Autodesk Fusion 360 part; units mm, degrees
(part 2 of 2)
  circle A962 centre (86.8214, 134.766) radius 1.25
  circle A963 centre (91.2857, 134.766) radius 1.25
  circle A964 centre (95.75, 134.766) radius 1.25
  circle A965 centre (100.2143, 134.766) radius 1.25
  circle A966 centre (104.6786, 134.766) radius 1.25
  circle A967 centre (109.1429, 134.766) radius 1.25
  circle A968 centre (113.6071, 134.766) radius 1.25
  circle A969 centre (118.0714, 134.766) radius 1.25
  circle A970 centre (122.5357, 134.766) radius 1.25
  circle A971 centre (127, 134.766) radius 1.25
  circle A972 centre (42.1786, 139.8723) radius 1.25
  circle A973 centre (46.6429, 139.8723) radius 1.25
  circle A974 centre (51.1071, 139.8723) radius 1.25
  circle A975 centre (55.5714, 139.8723) radius 1.25
  circle A976 centre (60.0357, 139.8723) radius 1.25
  circle A977 centre (64.5, 139.8723) radius 1.25
  circle A978 centre (68.9643, 139.8723) radius 1.25
  circle A979 centre (73.4286, 139.8723) radius 1.25
  circle A980 centre (77.8929, 139.8723) radius 1.25
  circle A981 centre (82.3571, 139.8723) radius 1.25
  circle A982 centre (86.8214, 139.8723) radius 1.25
  circle A983 centre (91.2857, 139.8723) radius 1.25
  circle A984 centre (95.75, 139.8723) radius 1.25
  circle A985 centre (100.2143, 139.8723) radius 1.25
  circle A986 centre (104.6786, 139.8723) radius 1.25
  circle A987 centre (109.1429, 139.8723) radius 1.25
  circle A988 centre (113.6071, 139.8723) radius 1.25
  circle A989 centre (118.0714, 139.8723) radius 1.25
  circle A990 centre (122.5357, 139.8723) radius 1.25
  circle A991 centre (127, 139.8723) radius 1.25
  circle A992 centre (42.1786, 144.9787) radius 1.25
  circle A993 centre (46.6429, 144.9787) radius 1.25
  circle A994 centre (51.1071, 144.9787) radius 1.25
  circle A995 centre (55.5714, 144.9787) radius 1.25
  circle A996 centre (60.0357, 144.9787) radius 1.25
  circle A997 centre (64.5, 144.9787) radius 1.25
  circle A998 centre (68.9643, 144.9787) radius 1.25
  circle A999 centre (73.4286, 144.9787) radius 1.25
  circle A1000 centre (77.8929, 144.9787) radius 1.25
  circle A1001 centre (82.3571, 144.9787) radius 1.25
  circle A1002 centre (86.8214, 144.9787) radius 1.25
  circle A1003 centre (91.2857, 144.9787) radius 1.25
  circle A1004 centre (95.75, 144.9787) radius 1.25
  circle A1005 centre (100.2143, 144.9787) radius 1.25
  circle A1006 centre (104.6786, 144.9787) radius 1.25
  circle A1007 centre (109.1429, 144.9787) radius 1.25
  circle A1008 centre (113.6071, 144.9787) radius 1.25
  circle A1009 centre (118.0714, 144.9787) radius 1.25
  circle A1010 centre (122.5357, 144.9787) radius 1.25
  circle A1011 centre (127, 144.9787) radius 1.25
  circle A1012 centre (42.1786, 150.0851) radius 1.25
  circle A1013 centre (46.6429, 150.0851) radius 1.25
  circle A1014 centre (51.1071, 150.0851) radius 1.25
  circle A1015 centre (55.5714, 150.0851) radius 1.25
  circle A1016 centre (60.0357, 150.0851) radius 1.25
  circle A1017 centre (64.5, 150.0851) radius 1.25
  circle A1018 centre (68.9643, 150.0851) radius 1.25
  circle A1019 centre (73.4286, 150.0851) radius 1.25
  circle A1020 centre (77.8929, 150.0851) radius 1.25
  circle A1021 centre (82.3571, 150.0851) radius 1.25
  circle A1022 centre (86.8214, 150.0851) radius 1.25
  circle A1023 centre (91.2857, 150.0851) radius 1.25
  circle A1024 centre (95.75, 150.0851) radius 1.25
  circle A1025 centre (100.2143, 150.0851) radius 1.25
  circle A1026 centre (104.6786, 150.0851) radius 1.25
  circle A1027 centre (109.1429, 150.0851) radius 1.25
  circle A1028 centre (113.6071, 150.0851) radius 1.25
  circle A1029 centre (118.0714, 150.0851) radius 1.25
  circle A1030 centre (122.5357, 150.0851) radius 1.25
  circle A1031 centre (127, 150.0851) radius 1.25
  circle A1032 centre (42.1786, 155.1915) radius 1.25
  circle A1033 centre (46.6429, 155.1915) radius 1.25
  circle A1034 centre (51.1071, 155.1915) radius 1.25
  circle A1035 centre (55.5714, 155.1915) radius 1.25
  circle A1036 centre (60.0357, 155.1915) radius 1.25
  circle A1037 centre (64.5, 155.1915) radius 1.25
  circle A1038 centre (68.9643, 155.1915) radius 1.25
  circle A1039 centre (73.4286, 155.1915) radius 1.25
  circle A1040 centre (77.8929, 155.1915) radius 1.25
  circle A1041 centre (82.3571, 155.1915) radius 1.25
  circle A1042 centre (86.8214, 155.1915) radius 1.25
  circle A1043 centre (91.2857, 155.1915) radius 1.25
  circle A1044 centre (95.75, 155.1915) radius 1.25
  circle A1045 centre (100.2143, 155.1915) radius 1.25
  circle A1046 centre (104.6786, 155.1915) radius 1.25
  circle A1047 centre (109.1429, 155.1915) radius 1.25
  circle A1048 centre (113.6071, 155.1915) radius 1.25
  circle A1049 centre (118.0714, 155.1915) radius 1.25
  circle A1050 centre (122.5357, 155.1915) radius 1.25
  circle A1051 centre (127, 155.1915) radius 1.25
  circle A1052 centre (42.1786, 160.2979) radius 1.25
  circle A1053 centre (46.6429, 160.2979) radius 1.25
  circle A1054 centre (51.1071, 160.2979) radius 1.25
  circle A1055 centre (55.5714, 160.2979) radius 1.25
  circle A1056 centre (60.0357, 160.2979) radius 1.25
  circle A1057 centre (64.5, 160.2979) radius 1.25
  circle A1058 centre (68.9643, 160.2979) radius 1.25
  circle A1059 centre (73.4286, 160.2979) radius 1.25
  circle A1060 centre (77.8929, 160.2979) radius 1.25
  circle A1061 centre (82.3571, 160.2979) radius 1.25
  circle A1062 centre (86.8214, 160.2979) radius 1.25
  circle A1063 centre (91.2857, 160.2979) radius 1.25
  circle A1064 centre (95.75, 160.2979) radius 1.25
  circle A1065 centre (100.2143, 160.2979) radius 1.25
  circle A1066 centre (104.6786, 160.2979) radius 1.25
  circle A1067 centre (109.1429, 160.2979) radius 1.25
  circle A1068 centre (113.6071, 160.2979) radius 1.25
  circle A1069 centre (118.0714, 160.2979) radius 1.25
  circle A1070 centre (122.5357, 160.2979) radius 1.25
  circle A1071 centre (127, 160.2979) radius 1.25
  circle A1072 centre (42.1786, 165.4043) radius 1.25
  circle A1073 centre (46.6429, 165.4043) radius 1.25
  circle A1074 centre (51.1071, 165.4043) radius 1.25
  circle A1075 centre (55.5714, 165.4043) radius 1.25
  circle A1076 centre (60.0357, 165.4043) radius 1.25
  circle A1077 centre (64.5, 165.4043) radius 1.25
  circle A1078 centre (68.9643, 165.4043) radius 1.25
  circle A1079 centre (73.4286, 165.4043) radius 1.25
  circle A1080 centre (77.8929, 165.4043) radius 1.25
  circle A1081 centre (82.3571, 165.4043) radius 1.25
  circle A1082 centre (86.8214, 165.4043) radius 1.25
  circle A1083 centre (91.2857, 165.4043) radius 1.25
  circle A1084 centre (95.75, 165.4043) radius 1.25
  circle A1085 centre (100.2143, 165.4043) radius 1.25
  circle A1086 centre (104.6786, 165.4043) radius 1.25
  circle A1087 centre (109.1429, 165.4043) radius 1.25
  circle A1088 centre (113.6071, 165.4043) radius 1.25
  circle A1089 centre (118.0714, 165.4043) radius 1.25
  circle A1090 centre (122.5357, 165.4043) radius 1.25
  circle A1091 centre (127, 165.4043) radius 1.25
  circle A1092 centre (42.1786, 170.5106) radius 1.25
  circle A1093 centre (46.6429, 170.5106) radius 1.25
  circle A1094 centre (51.1071, 170.5106) radius 1.25
  circle A1095 centre (55.5714, 170.5106) radius 1.25
  circle A1096 centre (60.0357, 170.5106) radius 1.25
  circle A1097 centre (64.5, 170.5106) radius 1.25
  circle A1098 centre (68.9643, 170.5106) radius 1.25
  circle A1099 centre (73.4286, 170.5106) radius 1.25
  circle A1100 centre (77.8929, 170.5106) radius 1.25
  circle A1101 centre (82.3571, 170.5106) radius 1.25
  circle A1102 centre (86.8214, 170.5106) radius 1.25
  circle A1103 centre (91.2857, 170.5106) radius 1.25
  circle A1104 centre (95.75, 170.5106) radius 1.25
  circle A1105 centre (100.2143, 170.5106) radius 1.25
  circle A1106 centre (104.6786, 170.5106) radius 1.25
  circle A1107 centre (109.1429, 170.5106) radius 1.25
  circle A1108 centre (113.6071, 170.5106) radius 1.25
  circle A1109 centre (118.0714, 170.5106) radius 1.25
  circle A1110 centre (122.5357, 170.5106) radius 1.25
  circle A1111 centre (127, 170.5106) radius 1.25
  circle A1112 centre (42.1786, 175.617) radius 1.25
  circle A1113 centre (46.6429, 175.617) radius 1.25
  circle A1114 centre (51.1071, 175.617) radius 1.25
  circle A1115 centre (55.5714, 175.617) radius 1.25
  circle A1116 centre (60.0357, 175.617) radius 1.25
  circle A1117 centre (64.5, 175.617) radius 1.25
  circle A1118 centre (68.9643, 175.617) radius 1.25
  circle A1119 centre (73.4286, 175.617) radius 1.25
  circle A1120 centre (77.8929, 175.617) radius 1.25
  circle A1121 centre (82.3571, 175.617) radius 1.25
  circle A1122 centre (86.8214, 175.617) radius 1.25
  circle A1123 centre (91.2857, 175.617) radius 1.25
  circle A1124 centre (95.75, 175.617) radius 1.25
  circle A1125 centre (100.2143, 175.617) radius 1.25
  circle A1126 centre (104.6786, 175.617) radius 1.25
  circle A1127 centre (109.1429, 175.617) radius 1.25
  circle A1128 centre (113.6071, 175.617) radius 1.25
  circle A1129 centre (118.0714, 175.617) radius 1.25
  circle A1130 centre (122.5357, 175.617) radius 1.25
  circle A1131 centre (127, 175.617) radius 1.25
  circle A1132 centre (42.1786, 180.7234) radius 1.25
  circle A1133 centre (46.6429, 180.7234) radius 1.25
  circle A1134 centre (51.1071, 180.7234) radius 1.25
  circle A1135 centre (55.5714, 180.7234) radius 1.25
  circle A1136 centre (60.0357, 180.7234) radius 1.25
  circle A1137 centre (64.5, 180.7234) radius 1.25
  circle A1138 centre (68.9643, 180.7234) radius 1.25
  circle A1139 centre (73.4286, 180.7234) radius 1.25
  circle A1140 centre (77.8929, 180.7234) radius 1.25
  circle A1141 centre (82.3571, 180.7234) radius 1.25
  circle A1142 centre (86.8214, 180.7234) radius 1.25
  circle A1143 centre (91.2857, 180.7234) radius 1.25
  circle A1144 centre (95.75, 180.7234) radius 1.25
  circle A1145 centre (100.2143, 180.7234) radius 1.25
  circle A1146 centre (104.6786, 180.7234) radius 1.25
  circle A1147 centre (109.1429, 180.7234) radius 1.25
  circle A1148 centre (113.6071, 180.7234) radius 1.25
  circle A1149 centre (118.0714, 180.7234) radius 1.25
  circle A1150 centre (122.5357, 180.7234) radius 1.25
  circle A1151 centre (127, 180.7234) radius 1.25
  circle A1152 centre (42.1786, 185.8298) radius 1.25
  circle A1153 centre (46.6429, 185.8298) radius 1.25
  circle A1154 centre (51.1071, 185.8298) radius 1.25
  circle A1155 centre (55.5714, 185.8298) radius 1.25
  circle A1156 centre (60.0357, 185.8298) radius 1.25
  circle A1157 centre (64.5, 185.8298) radius 1.25
  circle A1158 centre (68.9643, 185.8298) radius 1.25
  circle A1159 centre (73.4286, 185.8298) radius 1.25
  circle A1160 centre (77.8929, 185.8298) radius 1.25
  circle A1161 centre (82.3571, 185.8298) radius 1.25
  circle A1162 centre (86.8214, 185.8298) radius 1.25
  circle A1163 centre (91.2857, 185.8298) radius 1.25
  circle A1164 centre (95.75, 185.8298) radius 1.25
  circle A1165 centre (100.2143, 185.8298) radius 1.25
  circle A1166 centre (104.6786, 185.8298) radius 1.25
  circle A1167 centre (109.1429, 185.8298) radius 1.25
  circle A1168 centre (113.6071, 185.8298) radius 1.25
  circle A1169 centre (118.0714, 185.8298) radius 1.25
  circle A1170 centre (122.5357, 185.8298) radius 1.25
  circle A1171 centre (127, 185.8298) radius 1.25
  circle A1172 centre (42.1786, 190.9362) radius 1.25
  circle A1173 centre (46.6429, 190.9362) radius 1.25
  circle A1174 centre (51.1071, 190.9362) radius 1.25
  circle A1175 centre (55.5714, 190.9362) radius 1.25
  circle A1176 centre (60.0357, 190.9362) radius 1.25
  circle A1177 centre (64.5, 190.9362) radius 1.25
  circle A1178 centre (68.9643, 190.9362) radius 1.25
  circle A1179 centre (73.4286, 190.9362) radius 1.25
  circle A1180 centre (77.8929, 190.9362) radius 1.25
  circle A1181 centre (82.3571, 190.9362) radius 1.25
  circle A1182 centre (86.8214, 190.9362) radius 1.25
  circle A1183 centre (91.2857, 190.9362) radius 1.25
  circle A1184 centre (95.75, 190.9362) radius 1.25
  circle A1185 centre (100.2143, 190.9362) radius 1.25
  circle A1186 centre (104.6786, 190.9362) radius 1.25
  circle A1187 centre (109.1429, 190.9362) radius 1.25
  circle A1188 centre (113.6071, 190.9362) radius 1.25
  circle A1189 centre (118.0714, 190.9362) radius 1.25
  circle A1190 centre (122.5357, 190.9362) radius 1.25
  circle A1191 centre (127, 190.9362) radius 1.25
  circle A1192 centre (42.1786, 196.0426) radius 1.25
  circle A1193 centre (46.6429, 196.0426) radius 1.25
  circle A1194 centre (51.1071, 196.0426) radius 1.25
  circle A1195 centre (55.5714, 196.0426) radius 1.25
  circle A1196 centre (60.0357, 196.0426) radius 1.25
  circle A1197 centre (64.5, 196.0426) radius 1.25
  circle A1198 centre (68.9643, 196.0426) radius 1.25
  circle A1199 centre (73.4286, 196.0426) radius 1.25
  circle A1200 centre (77.8929, 196.0426) radius 1.25
  circle A1201 centre (82.3571, 196.0426) radius 1.25
  circle A1202 centre (86.8214, 196.0426) radius 1.25
  circle A1203 centre (91.2857, 196.0426) radius 1.25
  circle A1204 centre (95.75, 196.0426) radius 1.25
  circle A1205 centre (100.2143, 196.0426) radius 1.25
  circle A1206 centre (104.6786, 196.0426) radius 1.25
  circle A1207 centre (109.1429, 196.0426) radius 1.25
  circle A1208 centre (113.6071, 196.0426) radius 1.25
  circle A1209 centre (118.0714, 196.0426) radius 1.25
  circle A1210 centre (122.5357, 196.0426) radius 1.25
  circle A1211 centre (127, 196.0426) radius 1.25
  circle A1212 centre (42.1786, 201.1489) radius 1.25
  circle A1213 centre (46.6429, 201.1489) radius 1.25
  circle A1214 centre (51.1071, 201.1489) radius 1.25
  circle A1215 centre (55.5714, 201.1489) radius 1.25
  circle A1216 centre (60.0357, 201.1489) radius 1.25
  circle A1217 centre (64.5, 201.1489) radius 1.25
  circle A1218 centre (68.9643, 201.1489) radius 1.25
  circle A1219 centre (73.4286, 201.1489) radius 1.25
  circle A1220 centre (77.8929, 201.1489) radius 1.25
  circle A1221 centre (82.3571, 201.1489) radius 1.25
  circle A1222 centre (86.8214, 201.1489) radius 1.25
  circle A1223 centre (91.2857, 201.1489) radius 1.25
  circle A1224 centre (95.75, 201.1489) radius 1.25
  circle A1225 centre (100.2143, 201.1489) radius 1.25
  circle A1226 centre (104.6786, 201.1489) radius 1.25
  circle A1227 centre (109.1429, 201.1489) radius 1.25
  circle A1228 centre (113.6071, 201.1489) radius 1.25
  circle A1229 centre (118.0714, 201.1489) radius 1.25
  circle A1230 centre (122.5357, 201.1489) radius 1.25
  circle A1231 centre (127, 201.1489) radius 1.25
  circle A1232 centre (42.1786, 206.2553) radius 1.25
  circle A1233 centre (46.6429, 206.2553) radius 1.25
  circle A1234 centre (51.1071, 206.2553) radius 1.25
  circle A1235 centre (55.5714, 206.2553) radius 1.25
  circle A1236 centre (60.0357, 206.2553) radius 1.25
  circle A1237 centre (64.5, 206.2553) radius 1.25
  circle A1238 centre (68.9643, 206.2553) radius 1.25
  circle A1239 centre (73.4286, 206.2553) radius 1.25
  circle A1240 centre (77.8929, 206.2553) radius 1.25
  circle A1241 centre (82.3571, 206.2553) radius 1.25
  circle A1242 centre (86.8214, 206.2553) radius 1.25
  circle A1243 centre (91.2857, 206.2553) radius 1.25
  circle A1244 centre (95.75, 206.2553) radius 1.25
  circle A1245 centre (100.2143, 206.2553) radius 1.25
  circle A1246 centre (104.6786, 206.2553) radius 1.25
  circle A1247 centre (109.1429, 206.2553) radius 1.25
  circle A1248 centre (113.6071, 206.2553) radius 1.25
  circle A1249 centre (118.0714, 206.2553) radius 1.25
  circle A1250 centre (122.5357, 206.2553) radius 1.25
  circle A1251 centre (127, 206.2553) radius 1.25
  circle A1252 centre (42.1786, 211.3617) radius 1.25
  circle A1253 centre (46.6429, 211.3617) radius 1.25
  circle A1254 centre (51.1071, 211.3617) radius 1.25
  circle A1255 centre (55.5714, 211.3617) radius 1.25
  circle A1256 centre (60.0357, 211.3617) radius 1.25
  circle A1257 centre (64.5, 211.3617) radius 1.25
  circle A1258 centre (68.9643, 211.3617) radius 1.25
  circle A1259 centre (73.4286, 211.3617) radius 1.25
  circle A1260 centre (77.8929, 211.3617) radius 1.25
  circle A1261 centre (82.3571, 211.3617) radius 1.25
  circle A1262 centre (86.8214, 211.3617) radius 1.25
  circle A1263 centre (91.2857, 211.3617) radius 1.25
  circle A1264 centre (95.75, 211.3617) radius 1.25
  circle A1265 centre (100.2143, 211.3617) radius 1.25
  circle A1266 centre (104.6786, 211.3617) radius 1.25
  circle A1267 centre (109.1429, 211.3617) radius 1.25
  circle A1268 centre (113.6071, 211.3617) radius 1.25
  circle A1269 centre (118.0714, 211.3617) radius 1.25
  circle A1270 centre (122.5357, 211.3617) radius 1.25
  circle A1271 centre (127, 211.3617) radius 1.25
  circle A1272 centre (42.1786, 216.4681) radius 1.25
  circle A1273 centre (46.6429, 216.4681) radius 1.25
  circle A1274 centre (51.1071, 216.4681) radius 1.25
  circle A1275 centre (55.5714, 216.4681) radius 1.25
  circle A1276 centre (60.0357, 216.4681) radius 1.25
  circle A1277 centre (64.5, 216.4681) radius 1.25
  circle A1278 centre (68.9643, 216.4681) radius 1.25
  circle A1279 centre (73.4286, 216.4681) radius 1.25
  circle A1280 centre (77.8929, 216.4681) radius 1.25
  circle A1281 centre (82.3571, 216.4681) radius 1.25
  circle A1282 centre (86.8214, 216.4681) radius 1.25
  circle A1283 centre (91.2857, 216.4681) radius 1.25
  circle A1284 centre (95.75, 216.4681) radius 1.25
  circle A1285 centre (100.2143, 216.4681) radius 1.25
  circle A1286 centre (104.6786, 216.4681) radius 1.25
  circle A1287 centre (109.1429, 216.4681) radius 1.25
  circle A1288 centre (113.6071, 216.4681) radius 1.25
  circle A1289 centre (118.0714, 216.4681) radius 1.25
  circle A1290 centre (122.5357, 216.4681) radius 1.25
  circle A1291 centre (127, 216.4681) radius 1.25
  circle A1292 centre (42.1786, 221.5745) radius 1.25
  circle A1293 centre (46.6429, 221.5745) radius 1.25
  circle A1294 centre (51.1071, 221.5745) radius 1.25
  circle A1295 centre (55.5714, 221.5745) radius 1.25
  circle A1296 centre (60.0357, 221.5745) radius 1.25
  circle A1297 centre (64.5, 221.5745) radius 1.25
  circle A1298 centre (68.9643, 221.5745) radius 1.25
  circle A1299 centre (73.4286, 221.5745) radius 1.25
  circle A1300 centre (77.8929, 221.5745) radius 1.25
  circle A1301 centre (82.3571, 221.5745) radius 1.25
  circle A1302 centre (86.8214, 221.5745) radius 1.25
  circle A1303 centre (91.2857, 221.5745) radius 1.25
  circle A1304 centre (95.75, 221.5745) radius 1.25
  circle A1305 centre (100.2143, 221.5745) radius 1.25
  circle A1306 centre (104.6786, 221.5745) radius 1.25
  circle A1307 centre (109.1429, 221.5745) radius 1.25
  circle A1308 centre (113.6071, 221.5745) radius 1.25
  circle A1309 centre (118.0714, 221.5745) radius 1.25
  circle A1310 centre (122.5357, 221.5745) radius 1.25
  circle A1311 centre (127, 221.5745) radius 1.25
  circle A1312 centre (42.1786, 226.6809) radius 1.25
  circle A1313 centre (46.6429, 226.6809) radius 1.25
  circle A1314 centre (51.1071, 226.6809) radius 1.25
  circle A1315 centre (55.5714, 226.6809) radius 1.25
  circle A1316 centre (60.0357, 226.6809) radius 1.25
  circle A1317 centre (64.5, 226.6809) radius 1.25
  circle A1318 centre (68.9643, 226.6809) radius 1.25
  circle A1319 centre (73.4286, 226.6809) radius 1.25
  circle A1320 centre (77.8929, 226.6809) radius 1.25
  circle A1321 centre (82.3571, 226.6809) radius 1.25
  circle A1322 centre (86.8214, 226.6809) radius 1.25
  circle A1323 centre (91.2857, 226.6809) radius 1.25
  circle A1324 centre (95.75, 226.6809) radius 1.25
  circle A1325 centre (100.2143, 226.6809) radius 1.25
  circle A1326 centre (104.6786, 226.6809) radius 1.25
  circle A1327 centre (109.1429, 226.6809) radius 1.25
  circle A1328 centre (113.6071, 226.6809) radius 1.25
  circle A1329 centre (118.0714, 226.6809) radius 1.25
  circle A1330 centre (122.5357, 226.6809) radius 1.25
  circle A1331 centre (127, 226.6809) radius 1.25
  circle A1332 centre (42.1786, 231.7872) radius 1.25
  circle A1333 centre (46.6429, 231.7872) radius 1.25
  circle A1334 centre (51.1071, 231.7872) radius 1.25
  circle A1335 centre (55.5714, 231.7872) radius 1.25
  circle A1336 centre (60.0357, 231.7872) radius 1.25
  circle A1337 centre (64.5, 231.7872) radius 1.25
  circle A1338 centre (68.9643, 231.7872) radius 1.25
  circle A1339 centre (73.4286, 231.7872) radius 1.25
  circle A1340 centre (77.8929, 231.7872) radius 1.25
  circle A1341 centre (82.3571, 231.7872) radius 1.25
  circle A1342 centre (86.8214, 231.7872) radius 1.25
  circle A1343 centre (91.2857, 231.7872) radius 1.25
  circle A1344 centre (95.75, 231.7872) radius 1.25
  circle A1345 centre (100.2143, 231.7872) radius 1.25
  circle A1346 centre (104.6786, 231.7872) radius 1.25
  circle A1347 centre (109.1429, 231.7872) radius 1.25
  circle A1348 centre (113.6071, 231.7872) radius 1.25
  circle A1349 centre (118.0714, 231.7872) radius 1.25
  circle A1350 centre (122.5357, 231.7872) radius 1.25
  circle A1351 centre (127, 231.7872) radius 1.25
  circle A1352 centre (42.1786, 236.8936) radius 1.25
  circle A1353 centre (46.6429, 236.8936) radius 1.25
  circle A1354 centre (51.1071, 236.8936) radius 1.25
  circle A1355 centre (55.5714, 236.8936) radius 1.25
  circle A1356 centre (60.0357, 236.8936) radius 1.25
  circle A1357 centre (64.5, 236.8936) radius 1.25
  circle A1358 centre (68.9643, 236.8936) radius 1.25
  circle A1359 centre (73.4286, 236.8936) radius 1.25
  circle A1360 centre (77.8929, 236.8936) radius 1.25
  circle A1361 centre (82.3571, 236.8936) radius 1.25
  circle A1362 centre (86.8214, 236.8936) radius 1.25
  circle A1363 centre (91.2857, 236.8936) radius 1.25
  circle A1364 centre (95.75, 236.8936) radius 1.25
  circle A1365 centre (100.2143, 236.8936) radius 1.25
  circle A1366 centre (104.6786, 236.8936) radius 1.25
  circle A1367 centre (109.1429, 236.8936) radius 1.25
  circle A1368 centre (113.6071, 236.8936) radius 1.25
  circle A1369 centre (118.0714, 236.8936) radius 1.25
  circle A1370 centre (122.5357, 236.8936) radius 1.25
  circle A1371 centre (127, 236.8936) radius 1.25
  circle A1372 centre (42.1786, 242) radius 1.25
  circle A1373 centre (46.6429, 242) radius 1.25
  circle A1374 centre (51.1071, 242) radius 1.25
  circle A1375 centre (55.5714, 242) radius 1.25
  circle A1376 centre (60.0357, 242) radius 1.25
  circle A1377 centre (64.5, 242) radius 1.25
  circle A1378 centre (68.9643, 242) radius 1.25
  circle A1379 centre (73.4286, 242) radius 1.25
  circle A1380 centre (77.8929, 242) radius 1.25
  circle A1381 centre (82.3571, 242) radius 1.25
  circle A1382 centre (86.8214, 242) radius 1.25
  circle A1383 centre (91.2857, 242) radius 1.25
  circle A1384 centre (95.75, 242) radius 1.25
  circle A1385 centre (100.2143, 242) radius 1.25
  circle A1386 centre (104.6786, 242) radius 1.25
  circle A1387 centre (109.1429, 242) radius 1.25
  circle A1388 centre (113.6071, 242) radius 1.25
  circle A1389 centre (118.0714, 242) radius 1.25
  circle A1390 centre (122.5357, 242) radius 1.25
  circle A1391 centre (127, 242) radius 1.25
  dimension "d1" = 125
  dimension "d3" = 240
  dimension "d9" = 2
  dimension "d10" = 2
  dimension "d11" = 2.5
  dimension "d25" = 125
  dimension "d26" = 240
  constraint horizontal L0
  constraint vertical L1
  constraint horizontal L2
  constraint vertical L3
  constraint coincident L0.start L3.end
  constraint horizontal L4
  constraint vertical L5
  constraint horizontal L6
  constraint vertical L7
  constraint coincident L5.end L6.start
  measures "d1" distance of L0.start L0.end
  measures "d3" distance of L0.start L2.end
  measures "d9" distance of L0.start L4.end
  measures "d10" distance of L0.start L6.end
  measures "d11" diameter of A0
extrude "Extrude1" add sketch "Sketch1" along normal blind 5 contours L0 L1 L2 L3
equation "d1 = width"
equation "width = 125 mm"
equation "d3 = length"
equation "length = 240 mm"
equation "w_offset = 2 mm"
equation "l_offset = 2 mm"
equation "hole_size = 2.5 mm"
equation "d9 = w_offset"
equation "d10 = l_offset"
equation "d11 = hole_size"
equation "_l_MaxLength = length"
equation "_w_MaxLength = width"
equation "_l_NHoles = 48"
equation "_w_NHoles = 29"
equation "d23 = _w_NHoles"
equation "d24 = _l_NHoles"
equation "d25 = _w_MaxLength"
equation "d26 = _l_MaxLength"
equation "height = 5 mm"
equation "d28 = height"
equation "w_OUTPUTdbetweenholes = _w_MaxLength / _w_NHoles"
equation "l_OUTPUTdbetweenholes = _l_MaxLength / _w_NHoles"
